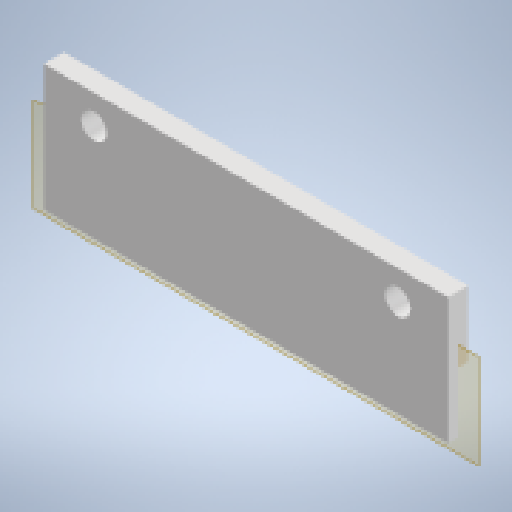
# Autodesk Inventor part: Adaptador
Saved by Autodesk Inventor 2023 (Build 270158000, 158)
## iProperties
Created: 2023-04-04
Part Number: Adaptador
Material: Genérico
Document SubType Name: Modeling
Designer: sergi
Density: 1 g/cm^3
Appearance: Valor por defecto
Author: sergi
Autodesk Inventor part; units mm, degrees
ref_plane "YZ Plane" through (0, 0, 0) normal (1, 0, 0) x (0, 1, 0)
ref_plane "XZ Plane" through (0, 0, 0) normal (0, 1, 0) x (-1, 0, 0)
ref_plane "XY Plane" through (0, 0, 0) normal (0, 0, 1) x (1, 0, 0)
ref_plane "Plano de trabajo1" through (0, 0, 0) normal (0, 0, 1) x (1, 0, 0)
sketch "Boceto1" plane through (0, 0, 0) normal (0, 0, 1) x (1, 0, 0)
  circle A0 centre (70, 9.3) radius 2.5 projected
  circle A1 centre (10, 9.3) radius 2.5 projected
  arc A2 (80, 12) -> (77, 15) centre (77, 12) ccw projected
  line L0 (3, 15) -> (77, 15) projected
  arc A3 (3, 15) -> (0, 12) centre (3, 12) ccw projected
  line L1 (0, 12) -> (0, -2) projected
  line L2 (0, -2) -> (0.1716, -2) projected
  arc A4 (3, 0) -> (0.1716, -2) centre (3, -3) ccw projected
  line L3 (77, 0) -> (3, 0) projected
  arc A5 (79.8284, -2) -> (77, 0) centre (77, -3) ccw projected
  line L4 (79.8284, -2) -> (80, -2) projected
  line L5 (80, -2) -> (80, 12) projected
  line L6 (0, 0) -> (80, 0)
  line L7 (80, 0) -> (80, 25)
  line L8 (80, 25) -> (0, 25)
  line L9 (0, 25) -> (0, 0)
  point P0 (0, 12)
  dimension "d0" = 25
  constraints: 8 end point, 2 parallel, 1 horizontal, 1 perpendicular
  measures "d0" distance of L7.end L6.end
extrude "Extrusión1" add sketch "Boceto1" along normal blind 2 contours A0 | A1 | L5 L6 L3 L1 A3 L0 A2 | A2 L0 A3 L9 L8 L7
sketch "Boceto2" plane through (0, 0, 0) normal (0, 0, -1) x (-1, 0, 0)
  circle A0 centre (-10, 9.3) radius 2.5 projected
  circle A1 centre (-70, 9.3) radius 2.5 projected
  line L0 (-10, 9.3) -> (-10, 19.3)
  line L1 (-70, 9.3) -> (-70, 19.3)
  point P0 (0, 0)
  dimension "d3" = 10
  dimension "d4" = 10
  constraints: 4 end point, 2 vertical
  measures "d3" distance of L0.start L0.end
  measures "d4" distance of L1.start L1.end
sketch "Boceto3" plane through (0, 0, 0) normal (0, 0, -1) x (-1, 0, 0)
  arc A0 (-77, 15) -> (-80, 12) centre (-77, 12) ccw projected
  line L0 (-80, -2) -> (-80, 12) projected
  line L1 (-80, -2) -> (0, -2) projected
  line L2 (0, -2) -> (0, 12) projected
  arc A1 (0, 12) -> (-3, 15) centre (-3, 12) ccw projected
  line L3 (-77, 15) -> (-3, 15) projected
  circle A2 centre (-70, 9.3) radius 2.5 projected
  circle A3 centre (-10, 9.3) radius 2.5 projected
  line L4 (-80, 25) -> (0, 25) projected
  line L5 (-80, 0) -> (-80, 25) projected
  line L6 (0, 0) -> (-80, 0) projected
  line L7 (0, 25) -> (0, 0) projected
  line L8 (-80, 25) -> (0, 25)
  line L9 (0, 25) -> (0, 15)
  line L10 (0, 15) -> (-80, 15)
  line L11 (-80, 15) -> (-80, 25)
  point P0 (-77, 15)
  point P1 (-3, 15)
  dimension "d14" = 10
  constraints: 8 end point, 2 parallel, 1 horizontal, 1 perpendicular, 1 point on line
  measures "d14" distance of L8.end L9.end
extrude "Extrusión2" add sketch "Boceto3" along normal blind 3 contours L10 L5 L4 L7 L3
hole "Agujero1" at (70, 19.3, 0) at (10, 19.3, 0) direction (0, 0, 1) diameter 5 end through all both
